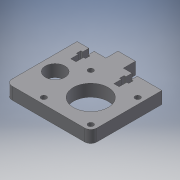
# Autodesk Inventor part: A8-0003
Saved by Autodesk Inventor 2016 SP2 (Build 200236200, 236)
## iProperties
Created: 2017-04-22
Part Number: A8-0003
Material: Generic
Document SubType Name: Modeling
Designer: EV
Density: 1 g/cm^3
Appearance: Default
Author: EV
Autodesk Inventor part; units mm, degrees
ref_plane "YZ Plane" through (0, 0, 0) normal (1, 0, 0) x (0, 1, 0)
ref_plane "XY Plane" through (0, 0, 0) normal (0, 0, 1) x (1, 0, 0)
sketch "Sketch1" plane through (0, 0, 0) normal (0, 1, 0) x (-1, 0, 0)
  line L0 (-4, 0) -> (-52, 0)
  line L1 (-56, -4) -> (-56, -47)
  line L2 (0, -47) -> (0, -4)
  line L3 (-19.75, -47) -> (-19.75, -55)
  line L4 (-19.75, -55) -> (-31.25, -55)
  line L5 (-31.25, -55) -> (-31.25, -47)
  line L6 (-7.75, -47) -> (-7.75, -43)
  line L7 (-7.75, -43) -> (-6.5, -43)
  line L8 (-6.5, -43) -> (-6.5, -40)
  line L9 (-6.5, -40) -> (-7.75, -40)
  line L10 (-7.75, -40) -> (-7.75, -35)
  line L11 (-7.75, -35) -> (-11.25, -35)
  line L12 (-11.25, -35) -> (-11.25, -40)
  line L13 (-11.25, -40) -> (-12.5, -40)
  line L14 (-12.5, -40) -> (-12.5, -43)
  line L15 (-12.5, -43) -> (-11.25, -43)
  line L16 (-11.25, -43) -> (-11.25, -47)
  line L17 (-36.25, -47) -> (-36.25, -43)
  line L18 (-36.25, -43) -> (-35, -43)
  line L19 (-35, -43) -> (-35, -40)
  line L20 (-35, -40) -> (-36.25, -40)
  line L21 (-36.25, -40) -> (-36.25, -35)
  line L22 (-36.25, -35) -> (-39.75, -35)
  line L23 (-39.75, -35) -> (-39.75, -40)
  line L24 (-39.75, -40) -> (-41, -40)
  line L25 (-41, -40) -> (-41, -43)
  line L26 (-41, -43) -> (-39.75, -43)
  line L27 (-39.75, -43) -> (-39.75, -47)
  line L28 (-19.75, -47) -> (-11.25, -47)
  line L29 (-7.75, -47) -> (0, -47)
  line L30 (-56, -47) -> (-39.75, -47)
  line L31 (-36.25, -47) -> (-31.25, -47)
  arc A0 (0, -4) -> (-4, 0) centre (-4, -4) ccw
  arc A1 (-52, 0) -> (-56, -4) centre (-52, -4) ccw
  point P0 (0, 0)
  point P1 (-56, 0)
  dimension "d0" = 56
  dimension "d1" = 47
  dimension "d2" = 8
  dimension "d3" = 11.5
  dimension "d4" = 19.75
  dimension "d5" = 4
  dimension "d6" = 3
  dimension "d7" = 5
  dimension "d8" = 3.5
  dimension "d9" = 6
  dimension "d10" = 7.75
  dimension "d11" = 3.5
  dimension "d12" = 6
  dimension "d13" = 16.25
  dimension "d14" = 4
  constraints: 64 end point, 23 perpendicular, 17 point on line, 6 parallel, 5 collinear, 5 equal length, 4 point on circle, 4 tangent, 2 centre point, 2 vertical, 1 equal radius, 1 horizontal
  measures "d0" distance of point (0, 0) point (-56, 0)
  measures "d1" distance of L2.start point (0, 0)
  measures "d2" distance of L3.start L3.end
  measures "d3" distance of L3.end L4.end
  measures "d4" distance between parallel lines of L3 L2
  measures "d5" distance of L6.start L6.end
  measures "d6" distance of L7.end L8.end
  measures "d7" distance of L9.end L10.end
  measures "d8" distance between parallel lines of L16 L6
  measures "d9" distance between parallel lines of L14 L8
  measures "d10" distance between parallel lines of L6 L2
  measures "d11" distance between parallel lines of L27 L17
  measures "d12" distance between parallel lines of L25 L19
  measures "d13" distance between parallel lines of L1 L27
  measures "d14" radius of A0
extrude "Extrusion1" add sketch "Sketch1" along normal blind 8
sketch "Sketch2" plane through (0, 8, 0) normal (0, 1, 0) x (1, 0, 0)
  line L0 (56, 4) -> (56, 47) construction
  line L1 (56, 47) -> (39.75, 47) construction
  line L2 (39.75, 47) -> (39.75, 43) construction
  line L3 (39.75, 43) -> (41, 43) construction
  line L4 (41, 43) -> (41, 40) construction
  line L5 (41, 40) -> (39.75, 40) construction
  line L6 (39.75, 40) -> (39.75, 35) construction
  line L7 (39.75, 35) -> (36.25, 35) construction
  line L8 (36.25, 35) -> (36.25, 40) construction
  line L9 (36.25, 40) -> (35, 40) construction
  line L10 (35, 40) -> (35, 43) construction
  line L11 (35, 43) -> (36.25, 43) construction
  line L12 (36.25, 43) -> (36.25, 47) construction
  line L13 (36.25, 47) -> (31.25, 47) construction
  line L14 (31.25, 47) -> (31.25, 55) construction
  line L15 (31.25, 55) -> (19.75, 55) construction
  line L16 (19.75, 55) -> (19.75, 47) construction
  line L17 (19.75, 47) -> (11.25, 47) construction
  line L18 (11.25, 47) -> (11.25, 43) construction
  line L19 (11.25, 43) -> (12.5, 43) construction
  line L20 (12.5, 43) -> (12.5, 40) construction
  line L21 (12.5, 40) -> (11.25, 40) construction
  line L22 (11.25, 40) -> (11.25, 35) construction
  line L23 (11.25, 35) -> (7.75, 35) construction
  line L24 (7.75, 35) -> (7.75, 40) construction
  line L25 (7.75, 40) -> (6.5, 40) construction
  line L26 (6.5, 40) -> (6.5, 43) construction
  line L27 (6.5, 43) -> (7.75, 43) construction
  line L28 (7.75, 43) -> (7.75, 47) construction
  line L29 (7.75, 47) -> (0, 47) construction
  line L30 (0, 47) -> (0, 4) construction
  arc A0 (0, 4) -> (4, 0) centre (4, 4) ccw construction
  line L31 (4, 0) -> (52, 0) construction
  arc A1 (52, 0) -> (56, 4) centre (52, 4) ccw construction
  line L32 (21, 4) -> (52, 4) construction
  line L33 (52, 4) -> (52, 35) construction
  line L34 (52, 35) -> (21, 35) construction
  line L35 (21, 35) -> (21, 4) construction
  line L36 (21, 35) -> (52, 4) construction
  point P0 (0, 0)
  point P1 (36.5, 19.5)
  point P2 (10, 22.5)
  dimension "d17" = 31
  dimension "d18" = 31
  dimension "d19" = 4
  dimension "d20" = 4
  dimension "d21" = 22.5
  dimension "d22" = 10
  constraints: 10 end point, 4 coincident, 2 parallel, 1 horizontal, 1 midpoint, 1 perpendicular
  measures "d17" distance of L32.start L32.end
  measures "d18" distance of L34.end L32.start
  measures "d19" distance between parallel lines of L31 L32
  measures "d20" distance between parallel lines of L0 L33
  measures "d21" distance from line of point (10, 22.5) L31
  measures "d22" distance from line of point (10, 22.5) L30
hole "Hole1" at (21, 8, -35) at (52, 8, -35) at (52, 8, -4) at (21, 8, -4) direction (0, -1, 0) diameter 3.5 end through all
hole "Hole2" at (36.5, 8, -19.5) direction (0, -1, 0) diameter 23 end through all
hole "Hole3" at (10, 8, -22.5) direction (0, -1, 0) diameter 13 end through all
ref_plane "Work Plane1" through (0, 4, 0) normal (0, 1, 0) x (-1, 0, 0)
equation "\"d11\" = d8"
equation "\"d12\" = d9"
equation "\"d44\" = 0.5 * THICKNESS"
equation "\"THICKNESS\" = 8"
body "Solid1"
